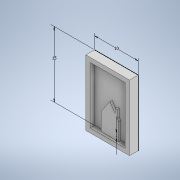
# Autodesk Inventor part: Painting
Saved by Autodesk Inventor 2022 (Build 260153000, 153)
## iProperties
Created: 2022-07-07
Part Number: Painting
Material: Generic
Document SubType Name: Modeling
Designer: mihir
Density: 1 g/cm^3
Appearance: Default
Author: mihir
Autodesk Inventor part; units mm, degrees
ref_plane "YZ Plane" through (0, 0, 0) normal (1, 0, 0) x (0, 1, 0)
ref_plane "XZ Plane" through (0, 0, 0) normal (0, 1, 0) x (-1, 0, 0)
ref_plane "XY Plane" through (0, 0, 0) normal (0, 0, 1) x (1, 0, 0)
sketch "Sketch1" plane through (0, 0, 0) normal (0, 0, 1) x (1, 0, 0)
  line L0 (0, 0) -> (10, 0)
  line L1 (10, 0) -> (10, 15)
  line L2 (10, 15) -> (0, 15)
  line L3 (0, 15) -> (0, 0)
  line L4 (9, 1) -> (1, 1)
  line L5 (1, 1) -> (1, 14)
  line L6 (1, 14) -> (9, 14)
  line L7 (9, 14) -> (9, 1)
  dimension "d0" = 10
  dimension "d1" = 15
  dimension "d2" = 1
  constraints: 16 end point, 4 parallel, 2 perpendicular, 1 horizontal, 3 other
  measures "d0" distance of L2.end L1.end
  measures "d1" distance of L2.end L0.start
  measures "d2" distance between parallel lines of L0 L4
extrude "Extrusion1" add sketch "Sketch1" along normal blind 1 contours L4 L5 L6 L7
sketch "Sketch2" plane through (0, 0, 0) normal (0, 0, -1) x (-1, 0, 0)
  line L0 (-1, 1) -> (-9, 1) projected
  line L1 (-9, 14) -> (-1, 14) projected
  line L2 (-9, 1) -> (-1, 1)
  line L3 (-1, 1) -> (-1, 14)
  line L4 (-1, 14) -> (-9, 14)
  line L5 (-9, 14) -> (-9, 1)
  point P0 (0, 0)
  constraints: 8 end point, 2 parallel, 1 horizontal, 1 perpendicular
extrude "Extrusion2" add sketch "Sketch1" along normal blind 2
sketch "Sketch3" plane through (0, 0, 1) normal (0, 0, 1) x (1, 0, 0)
  line L0 (9, 1) -> (1, 1) projected
  line L1 (3, 1) -> (7, 1)
  line L2 (7, 1) -> (7, 5)
  line L3 (7, 5) -> (3, 5)
  line L4 (3, 5) -> (3, 1)
  line L5 (9, 14) -> (9, 1) projected
  line L6 (3, 5) -> (7, 5)
  line L7 (7, 5) -> (5, 8)
  line L8 (5, 8) -> (3, 5)
  line L9 (6.1824, 6.2265) -> (6.1824, 7.2265)
  line L10 (6.1824, 7.2265) -> (6.6824, 7.2265)
  line L11 (6.6824, 7.2265) -> (6.6824, 5.4765)
  point P0 (0, 0)
  dimension "d7" = 4
  dimension "d8" = 4
  dimension "d9" = 2
  dimension "d10" = 3
  dimension "d11" = 1
  dimension "d12" = 0.5
  constraints: 20 end point, 3 perpendicular, 3 point on line, 2 horizontal, 2 parallel, 1 equal length, 1 vertical
  measures "d7" distance of L3.end L2.end
  measures "d8" distance of L1.end L2.end
  measures "d9" distance between parallel lines of L5 L2
  measures "d10" distance from line of L3 L7.end
  measures "d11" distance of L9.start L9.end
  measures "d12" distance of L9.end L10.end
extrude "Extrusion3" add sketch "Sketch3" along normal blind 0.5
body "Solid1"
